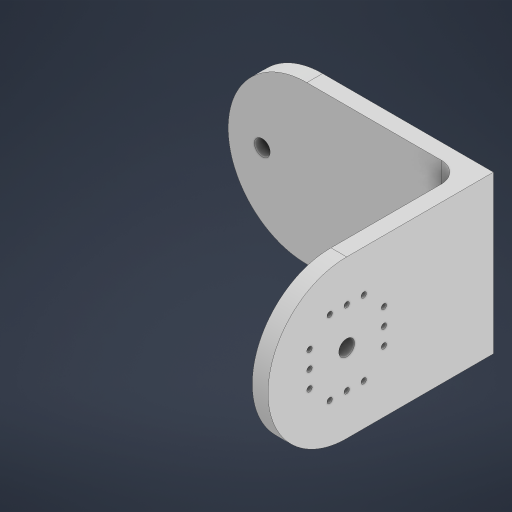
# Autodesk Inventor part: acople_1
Saved by Autodesk Inventor 2023.1 (Build 271208000, 208)
## iProperties
Created: 2022-10-22
Part Number: acople_1
Material: Generic
Document SubType Name: Modeling
Designer: amtat
Density: 1 g/cm^3
Appearance: Default
Author: amtat
Autodesk Inventor part; units mm, degrees
ref_plane "YZ Plane" through (0, 0, 0) normal (1, 0, 0) x (0, 1, 0)
ref_plane "XZ Plane" through (0, 0, 0) normal (0, 1, 0) x (-1, 0, 0)
ref_plane "XY Plane" through (0, 0, 0) normal (0, 0, 1) x (1, 0, 0)
sketch "Sketch1" plane through (0, 0, 0) normal (0, 0, 1) x (1, 0, 0)
  line L0 (0, 0) -> (46.2, 0)
  line L1 (46.2, 0) -> (46.2, 30)
  line L2 (46.2, 30) -> (0, 30)
  line L3 (0, 30) -> (0, 0)
  dimension "d0" = 46.2
  dimension "d1" = 30
  constraints: 8 end point, 2 perpendicular, 1 horizontal, 1 vertical
  measures "d0" distance of L0.start L0.end
  measures "d1" distance of L0.end L1.end
extrude "Extrusion1" add sketch "Sketch1" along normal blind 3
sketch "Sketch2" plane through (0, 0, 3) normal (0, 0, 1) x (1, 0, 0)
  line L0 (0, 0) -> (46.2, 0) projected
  line L1 (0, 0) -> (0, 15)
  line L2 (0, 30) -> (0, 0) projected
  line L3 (0, 15) -> (23.1, 15)
  line L4 (46.2, 0) -> (46.2, 30) projected
  line L5 (23.1, 15) -> (38.1, 15)
  line L6 (23.1, 15) -> (8.1, 15)
  circle A0 centre (8.1, 15) radius 1.5
  circle A1 centre (38.1, 15) radius 1.5
  dimension "d4" = 15
  dimension "d5" = 23.1
  dimension "d6" = 15
  dimension "d7" = 15
  dimension "d8" = 3
  dimension "d9" = 3
  constraints: 8 end point, 2 centre point, 2 coincident, 1 horizontal, 1 midpoint, 1 perpendicular, 1 point on line
  measures "d4" distance of L0.start L1.end
  measures "d5" distance of L1.end L3.end
  measures "d6" distance of L3.end L5.end
  measures "d7" distance of L3.end L6.end
  measures "d8" diameter of A0
  measures "d9" diameter of A1
extrude "Extrusion2" cut sketch "Sketch2" against normal blind 3
sketch "Sketch3" plane through (0, 0, 3) normal (0, 0, 1) x (1, 0, 0)
  circle A0 centre (38.1, 15) radius 1.5 projected
  circle A1 centre (8.1, 15) radius 1.5 projected
  line L0 (46.2, 0) -> (46.2, 30) projected
  line L1 (46.2, 30) -> (0, 30) projected
  line L2 (0, 30) -> (0, 0) projected
  line L3 (0, 0) -> (46.2, 0) projected
  circle A2 centre (38.1, 15) radius 3.5
  line L4 (38.1, 15) -> (41.6, 15)
  line L5 (41.6, 15) -> (42.6, 15)
  line L6 (42.6, 15) -> (45.6, 15)
  line L7 (45.6, 15) -> (45.6, 30)
  line L8 (45.6, 15) -> (45.6, 0)
  line L9 (0, 0) -> (46.2, 0) projected
  line L10 (45.6, 0) -> (46.2, 0)
  circle A3 centre (8.1, 15) radius 3.5
  line L11 (8.1, 15) -> (4.6, 15)
  line L12 (4.6, 15) -> (1.6, 15)
  line L13 (1.6, 15) -> (1.6, 30)
  line L14 (46.2, 30) -> (0, 30) projected
  line L15 (1.6, 30) -> (0, 30)
  line L16 (1.6, 15) -> (1.6, 0)
  dimension "d12" = 7
  dimension "d17" = 7
  dimension "d13" = 1
  dimension "d14" = 3
  dimension "d15" = 15
  dimension "d16" = 15
  dimension "d18" = 3
  constraints: 22 end point, 8 point on line, 2 coincident, 2 collinear, 2 horizontal alignment, 1 horizontal, 1 perpendicular, 4 other
  measures "d13" distance of L4.end L5.end
  measures "d14" distance of L5.end L6.end
  measures "d15" distance of L6.end L7.end
  measures "d16" distance of L6.end L8.end
  measures "d18" distance of L11.end L12.end
extrude "Extrusion6" cut sketch "Sketch3" against normal blind 40 contours L3 L2 L1 L13 L16
sketch "Sketch6" plane through (0, 0, 3) normal (0, 0, 1) x (1, 0, 0)
  line L0 (1.6, 30) -> (1.6, 0) projected
  line L1 (1.6, 0) -> (46.2, 0) projected
  line L2 (46.2, 0) -> (46.2, 30) projected
  line L3 (46.2, 30) -> (1.6, 30) projected
  circle A0 centre (8.1, 15) radius 1.5 projected
  circle A1 centre (38.1, 15) radius 1.5 projected
  line L4 (1.6, 0) -> (46.2, 0) projected
  line L5 (46.2, 0) -> (49.2, 0)
  line L6 (49.2, 0) -> (49.2, 30)
  line L7 (49.2, 30) -> (46.2, 30)
  point P0 (0, 0)
  dimension "d33" = 3
  dimension "d34" = 30
  constraints: 6 end point, 1 horizontal, 1 perpendicular
  measures "d33" distance of L1.end L5.end
  measures "d34" distance of L5.end L6.end
extrude "Extrusion7" add sketch "Sketch6" against normal blind 3 contours L7 L6 L5 L2
sketch "Sketch7" plane through (0, 0, 3) normal (0, 0, 1) x (1, 0, 0)
  line L0 (1.6, 30) -> (1.6, 0) projected
  line L1 (1.6, 0) -> (49.2, 0) projected
  line L2 (49.2, 0) -> (49.2, 30) projected
  line L3 (49.2, 30) -> (1.6, 30) projected
  circle A0 centre (8.1, 15) radius 1.5 projected
  circle A1 centre (38.1, 15) radius 1.5 projected
  line L4 (49.2, 30) -> (49.2, 0) projected
  line L5 (49.2, 0) -> (46.2, 0)
  line L6 (1.6, 0) -> (49.2, 0) projected
  line L7 (46.2, 0) -> (46.2, 30)
  line L8 (49.2, 30) -> (1.6, 30) projected
  line L9 (46.2, 30) -> (49.2, 30)
  point P0 (0, 0)
  dimension "d37" = 3
  constraints: 6 end point, 2 point on line, 1 collinear, 1 perpendicular
  measures "d37" distance of L1.end L5.end
extrude "Extrusion8" add sketch "Sketch7" along normal blind 40 contours L3 L2 L1 L7
sketch "Sketch8" plane through (46.2, 0, 3) normal (-1, 0, 0) x (0, 0, 1)
  line L0 (0, 0) -> (0, 30) projected
  line L1 (0, 0) -> (40, 0) projected
  line L2 (40, 30) -> (40, 0) projected
  line L3 (0, 30) -> (40, 30) projected
  line L4 (0, 30) -> (0, 15)
  line L5 (0, 30) -> (0, 0) projected
  line L6 (0, 15) -> (25, 15)
  circle A0 centre (25, 15) radius 1.5
  circle A1 centre (25, 15) radius 15
  line L7 (-3, 30) -> (40, 30) projected
  line L8 (40, 0) -> (-3, 0) projected
  point P0 (25, 30)
  point P1 (25, 0)
  point P2 (40, 15)
  point P3 (25, 0)
  point P4 (25, 30)
  dimension "d40" = 15
  dimension "d41" = 25
  dimension "d42" = 3
  constraints: 4 end point, 2 centre point, 2 coincident, 2 point on circle, 2 point on line, 1 midpoint, 1 perpendicular
  measures "d40" distance of L0.end L4.end
  measures "d41" distance of L4.end L6.end
  measures "d42" diameter of A0
extrude "Extrusion9" cut sketch "Sketch8" against normal blind 40 contours A1 L2 L1 | A1 L3 L2 | A0
fillet "Fillet1" radius 4 1 edges at (46.2, 15, 3)
fillet "Fillet2" radius 15 2 edges at (1.6, 30, 1.5) (1.6, 0, 1.5)
sketch "Sketch9" plane through (46.2, 15, 28) normal (-1, 0, 0) x (0, 0, 1)
  line L0 (-21, -15) -> (-21, 15) projected
  line L1 (-21, -15) -> (0, -15) projected
  arc A0 (0, -15) -> (0, 15) centre (0, 0) ccw projected
  line L2 (-21, 15) -> (0, 15) projected
  circle A1 centre (0, 0) radius 1.5 projected
  line L3 (0, 0) -> (0, 7.1)
  line L4 (0, 7.1) -> (3.25, 7.1)
  line L5 (0, 7.1) -> (-3.25, 7.1)
  circle A2 centre (0, 7.1) radius 0.5
  circle A3 centre (3.25, 7.1) radius 0.5
  circle A4 centre (-3.25, 7.1) radius 0.5
  line L6 (0, 0) -> (4.7365, 0)
  line L7 (0, 0) -> (5.6569, 5.6569)
  line L8 (0, 0) -> (8, 0) construction
  circle A5 centre (0, -7.1) radius 0.5
  circle A6 centre (3.25, -7.1) radius 0.5
  circle A7 centre (-3.25, -7.1) radius 0.5
  circle A8 centre (7.1, 0) radius 0.5
  circle A9 centre (7.1, 3.25) radius 0.5
  circle A10 centre (7.1, -3.25) radius 0.5
  circle A11 centre (-7.1, -3.25) radius 0.5
  circle A12 centre (-7.1, 0) radius 0.5
  circle A13 centre (-7.1, 3.25) radius 0.5
  point P0 (-28, -15)
  dimension "d47" = 7.1
  dimension "d48" = 3.25
  dimension "d49" = 3.25
  dimension "d50" = 1
  dimension "d51" = 1
  dimension "d52" = 1
  dimension "d53" = 8
  dimension "d54" = 45
  constraints: 12 centre point, 12 end point, 9 symmetric about line, 4 horizontal, 3 coincident, 1 equal length, 1 vertical, 9 other
  measures "d47" distance of L3.start L3.end
  measures "d48" distance of L3.end L4.end
  measures "d49" distance of L3.end L5.end
  measures "d50" diameter of A2
  measures "d51" diameter of A3
  measures "d52" diameter of A4
  measures "d53" distance of L3.start L7.end
  measures "d54" angle of L8 L7
extrude "Extrusion10" cut sketch "Sketch9" against normal blind 40 contours A2 L5 L3 | L3 L4 A2 | L5 A2 L4 | A3 | A4 | A5 | A6 | A7 | A8 | A9 | A10 | A11 | A12 | A13
body "Solid1"
